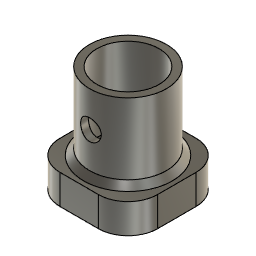
cube_twister_printer v2 (Autodesk Fusion 360 design; units mm, degrees)
Autodesk Fusion 360 part; units mm, degrees
sketch "Sketch1" plane through (0, 0, 0) normal (0, 0, 1) x (1, 0, 0)
  circle A0 centre (0, 0) radius 5.25
  circle A1 centre (0, 0) radius 6.5
  dimension "d1" = 10.5
  dimension "d2" = 1.25
  constraint coincident A0.centre A1.centre
  measures "d1" diameter of A0
sketch "Sketch2" plane through (0, 0, 0) normal (0, 0, 1) x (1, 0, 0)
  arc A0 (3.25, -8.25) -> (8.25, -3.25) centre (3.25, -3.25) ccw
  line L0 (3.25, 7.05) -> (-3.25, 7.05)
  line L1 (-8.25, 8.25) -> (8.25, -8.25) construction
  line L2 (8.25, -3.25) -> (8.25, 3.25)
  line L3 (7.05, -3.25) -> (7.05, 3.25)
  circle A1 centre (0, 0) radius 5.5
  arc A2 (-3.25, 8.25) -> (-8.25, 3.25) centre (-3.25, 3.25) ccw
  line L4 (8.25, 8.25) -> (-8.25, -8.25) construction
  line L5 (-8.25, 3.25) -> (-8.25, -3.25)
  arc A3 (-7.05, -3.25) -> (-3.25, -7.05) centre (-3.25, -3.25) ccw
  line L6 (3.25, 9.25) -> (-3.25, 9.25)
  arc A4 (-8.25, -3.25) -> (-3.25, -8.25) centre (-3.25, -3.25) ccw
  line L7 (-3.25, -7.05) -> (3.25, -7.05)
  arc A5 (8.25, 3.25) -> (3.25, 8.25) centre (3.25, 3.25) ccw
  arc A6 (3.25, -9.25) -> (9.25, -3.25) centre (3.25, -3.25) ccw
  line L8 (3.25, 8.25) -> (-3.25, 8.25)
  line L9 (9.25, -3.25) -> (9.25, 3.25)
  arc A7 (3.25, -7.05) -> (7.05, -3.25) centre (3.25, -3.25) ccw
  arc A8 (-3.25, 7.05) -> (-7.05, 3.25) centre (-3.25, 3.25) ccw
  arc A9 (-9.25, -3.25) -> (-3.25, -9.25) centre (-3.25, -3.25) ccw
  circle A10 centre (0, 0) radius 4.5
  line L10 (-3.25, -9.25) -> (3.25, -9.25)
  arc A11 (7.05, 3.25) -> (3.25, 7.05) centre (3.25, 3.25) ccw
  line L11 (-9.25, 3.25) -> (-9.25, -3.25)
  arc A12 (9.25, 3.25) -> (3.25, 9.25) centre (3.25, 3.25) ccw
  line L12 (-3.25, -8.25) -> (3.25, -8.25)
  arc A13 (-3.25, 9.25) -> (-9.25, 3.25) centre (-3.25, 3.25) ccw
  line L13 (-7.05, 3.25) -> (-7.05, -3.25)
  dimension "d3" = 1
  dimension "d4" = 1.2
  dimension "d5" = 1
  dimension "d6" = 16.5
  dimension "d7" = 16.5
  dimension "d8" = 5
  dimension "d9" = 11
  constraint horizontal L8
  constraint perpendicular L5 L8
  constraint parallel L8 L12
  constraint parallel L2 L5
  constraint coincident A1.centre L4
  constraint coincident A1.centre L1
  constraint coincident A1.centre A10.centre
  constraint coincident L1.start L5
  constraint coincident L1.start L8
  constraint tangent A2 L5
  constraint tangent A2 L8
  constraint coincident L4.start L2
  constraint coincident L4.start L8
  constraint tangent L2 A5
  constraint tangent A5 L8
  constraint equal A2 A5
  constraint coincident L1.end L12
  constraint coincident L1.end L2
  constraint tangent A0 L12
  constraint tangent A0 L2
  constraint equal A0 A2
  constraint coincident L4.end L12
  constraint coincident L4.end L5
  constraint tangent A4 L12
  constraint tangent L5 A4
  constraint equal A2 A4
  measures "d6" distance of L1.end L4.end
  measures "d7" distance of L1.start L4.end
  measures "d8" radius of A2
  measures "d9" diameter of A1
extrude "Extrude1" add sketch "Sketch2" along normal blind 5 contours A0 L2 A2 L5 A4 A5 L8 L12 | A1 makes body 1 at (7.45, 1.0833, 0) makes body 2 at (5.4932, -0.2742, 3.3333)
extrude "Extrude2" add sketch "Sketch2" against normal blind 1 from surface at 5 contours A0 L2 A2 L5 A4 A5 L8 L12 | L0 L3 A3 L7 A7 A8 A11 L13 | A1 | A10 bodies 1 2
extrude "Extrude3" add sketch "Sketch1" along normal blind 13 from surface at 5 bodies 1
ref_plane "WorkPlane1" through (0, -6.5, 9.9379) normal (0, -1, 0) x (-1, 0, 0)
sketch "Sketch3" plane through (0, -6.5, 0) normal (0, -1, 0) x (-1, 0, 0)
  line L0 (0, 0) -> (0, -19) construction
  line L1 (0, 0) -> (0, -5) construction
  line L2 (0, -5) -> (0, -19) construction
  circle A0 centre (0, -12) radius 1.75
  dimension "d19" = 19
  dimension "d20" = 5
  dimension "d21" = 3.5
  constraint coincident L0.start L1.start
  constraint vertical L0
  constraint coincident L0 L1.end
  constraint midpoint L2 A0.centre
  measures "d19" distance of L0.start L0.end
  measures "d20" distance of L0.start L1.end
  measures "d21" diameter of A0
extrude "Extrude4" cut sketch "Sketch3" against normal blind 4 bodies 1
chamfer "Chamfer1" distance 1 angle 45 1 edges at (-6.0601, 2.3505, 5) on bodies 1
chamfer "Chamfer2" distance 1 angle 45 8 edges at (5.937, -5.937, 4) (7.05, 0, 4) (5.937, 5.937, 4) (0, 7.05, 4) (-5.937, 5.937, 4) (-7.05, 0, 4) (-5.937, -5.937, 4) (0, -7.05, 4) on bodies 1
named bodies: "cube_twister_printer"
